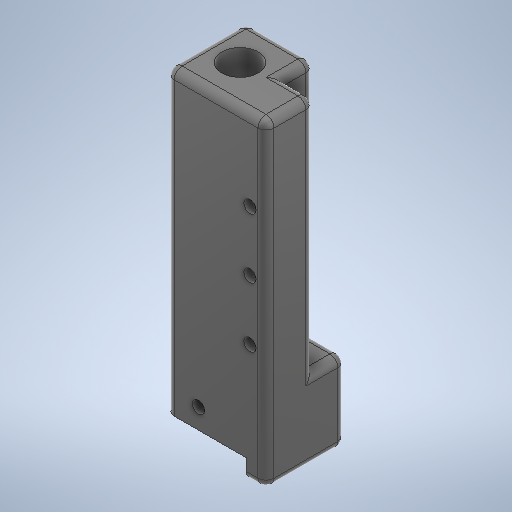
# Autodesk Inventor part: finger2
Saved by Autodesk Inventor 2026.2 (Build 302298010, 298A)
## iProperties
Created: 2026-05-11
Part Number: finger2
Material: ABS Plastic
Document SubType Name: Modeling
Designer: chris
Density: 1.06 g/cm^3
Appearance: Smooth - White
Author: chris
Autodesk Inventor part; units mm, degrees
ref_plane "YZ Plane" through (0, 0, 0) normal (1, 0, 0) x (0, 1, 0)
ref_plane "XZ Plane" through (0, 0, 0) normal (0, 1, 0) x (-1, 0, 0)
ref_plane "XY Plane" through (0, 0, 0) normal (0, 0, 1) x (1, 0, 0)
sketch "Sketch1" plane through (0, 0, 0) normal (0, 1, 0) x (-1, 0, 0)
  line L0 (10, 10) -> (-10, 10)
  line L1 (-10, 10) -> (-10, -10)
  line L2 (-10, -10) -> (10, -10)
  line L3 (10, -10) -> (10, 10)
  line L4 (10, 10) -> (-10, -10) construction
  line L5 (-10, 10) -> (10, -10) construction
  point P0 (0, 0)
  dimension "d0" = 20
  dimension "d1" = 20
  constraints: 12 end point, 2 midpoint, 2 parallel, 1 horizontal, 1 perpendicular
  measures "d0" distance of L2.end L1.end
  measures "d1" distance of L1.end L0.end
extrude "Extrusion1" add sketch "Sketch1" along normal blind 75
sketch "Sketch2" plane through (0, 75, 0) normal (0, 1, 0) x (1, 0, 0)
  circle A0 centre (-1.5, 0) radius 4.6
  line L0 (-10, -10) -> (10, -10) projected
  line L1 (-10, 10) -> (-10, -10) projected
  dimension "d4" = 9.2
  dimension "d25" = 10
  dimension "d26" = 8.5
  constraints: 1 centre point, 1 coincident
  measures "d4" diameter of A0
  measures "d25" distance from line of L0 point (-1.5, 0)
  measures "d26" distance from line of L1 point (-1.5, 0)
extrude "Extrusion2" cut sketch "Sketch2" against normal blind 10
sketch "Sketch3" plane through (0, 0, 0) normal (0, -1, 0) x (1, 0, 0)
  circle A0 centre (-1.5, 0) radius 7.5
  line L0 (10, -10) -> (-10, -10) projected
  line L1 (-10, -10) -> (-10, 10) projected
  dimension "d7" = 15
  dimension "d27" = 10
  dimension "d28" = 8.5
  constraints: 1 centre point, 1 coincident
  measures "d7" diameter of A0
  measures "d27" distance from line of point (-1.5, 0) L0
  measures "d28" distance from line of L1 point (-1.5, 0)
extrude "Extrusion3" cut sketch "Sketch3" against normal blind 65
sketch "Sketch5" plane through (10, 0, 10) normal (1, 0, 0) x (0, 0, -1)
  line L0 (20, 75) -> (0, 75)
  line L1 (0, 75) -> (0, 0)
  line L2 (0, 0) -> (20, 0)
  line L3 (20, 0) -> (20, 75)
  line L4 (20, 0) -> (20, 75) projected
  line L5 (0, 0) -> (20, 0) projected
  line L6 (0, 75) -> (20, 75) projected
  line L7 (0, 0) -> (0, 75) projected
  point P0 (10, 0)
  constraints: 8 end point, 4 collinear, 2 parallel, 1 horizontal, 1 perpendicular
extrude "Extrusion5" add sketch "Sketch5" along normal blind 5
sketch "Sketch7" plane through (-10, 0, -10) normal (0, 0, -1) x (-1, 0, 0)
  circle A0 centre (-21, 55) radius 1.55
  circle A1 centre (-21, 40) radius 1.55
  circle A2 centre (-21, 25) radius 1.55
  line L0 (0, 75) -> (-25, 75) projected
  line L1 (-25, 0) -> (-25, 75) projected
  point P0 (-10, 0)
  dimension "d16" = 3.1
  dimension "d17" = 3.1
  dimension "d18" = 3.1
  dimension "d19" = 20
  dimension "d20" = 15
  dimension "d21" = 15
  dimension "d22" = 4
  constraints: 3 centre point, 2 vertical alignment
  measures "d16" diameter of A0
  measures "d17" diameter of A1
  measures "d18" diameter of A2
  measures "d19" distance from line of L0 A0.centre
  measures "d20" distance of A0.centre A1.centre
  measures "d21" distance of A1.centre A2.centre
  measures "d22" distance from line of L1 A0.centre
extrude "Extrusion6" cut sketch "Sketch7" against normal blind 20
sketch "Sketch8" plane through (-10, 0, -10) normal (0, 0, -1) x (-1, 0, 0)
  line L0 (-17, 75) -> (-25, 75)
  line L1 (-25, 75) -> (-25, 15)
  line L2 (-25, 15) -> (-17, 15)
  line L3 (-17, 15) -> (-17, 75)
  line L4 (0, 0) -> (-25, 0) projected
  line L5 (0, 75) -> (-25, 75) projected
  line L6 (-25, 0) -> (-25, 75) projected
  point P0 (-10, 0)
  dimension "d29" = 8
  dimension "d32" = 15
  constraints: 8 end point, 2 collinear, 2 parallel, 1 horizontal, 1 perpendicular
  measures "d29" distance of L1.end L2.end
  measures "d32" distance between parallel lines of L4 L2
extrude "Extrusion7" cut sketch "Sketch8" against normal blind 8
sketch "Sketch9" plane through (-10, 0, -10) normal (0, 0, -1) x (-1, 0, 0)
  circle A0 centre (-8.1, 5) radius 1.55
  line L0 (0, 0) -> (0, 75) projected
  line L1 (0, 0) -> (-25, 0) projected
  point P0 (-10, 0)
  dimension "d33" = 3.1
  dimension "d34" = 8.1
  dimension "d35" = 5
  constraints: 1 centre point
  measures "d33" diameter of A0
  measures "d34" distance from line of L0 A0.centre
  measures "d35" distance from line of L1 A0.centre
extrude "Extrusion8" cut sketch "Sketch9" against normal through all
sketch "Sketch10" plane through (0, 0, 0) normal (0, -1, 0) x (1, 0, 0)
  line L0 (15, -10) -> (10, -10)
  line L1 (10, -10) -> (10, 10)
  line L2 (10, 10) -> (15, 10)
  line L3 (15, 10) -> (15, -10)
  line L4 (-10, -10) -> (15, -10) projected
  line L5 (-10, 10) -> (15, 10) projected
  line L6 (15, 10) -> (15, -10) projected
  point P0 (0, 0)
  dimension "d38" = 5
  constraints: 8 end point, 3 collinear, 2 parallel, 1 horizontal, 1 perpendicular
  measures "d38" distance of L1.end L2.end
extrude "Extrusion9" add sketch "Sketch10" along normal blind 5
fillet "Fillet1" radius 2 17 edges at (15, 35, 10) (-10, 37.5, 10) (15, 45, -2) (7, 45, -10) (-10, 37.5, -10) (-1.5, 75, -10) (7, 75, -6) (11, 75, -2) (15, 75, 4) (2.5, 75, 10) (-10, 75, 0) (11, 15, -10) (15, 15, -6) (15, 5, -10) (15, -5, 0) (12.5, -5, -10) (12.5, -5, 10)
body "Solid1"
